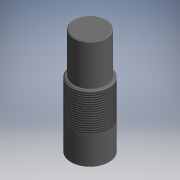
# Autodesk Inventor part: ESBF-BS-100-ESBF-BS-100---(KSA)
Saved by Autodesk Inventor 2017.3 (Build 213256000, 256)
## iProperties
Part Number: ESBF-BS-100-ESBF-BS-100---(KSA)
Material: Generic
Catalog Web Link: www.cadenas.de
Description: ESBF-(KSA)-Electro-cylinder
Vendor: FESTO
Document SubType Name: Modeling
Designer: partserver
Manufacturer: FESTO
Mass: 43.39 g
Surface Area: 76.8882 cm^2
Volume: 43.39 cm^3
Density: 1 g/cm^3
Appearance: PSOLRGB-128-128-128
Category: PARTsolutions
Company: FESTO
Title: ESBF-BS-100-ESBF-BS-100---(KSA)
Author: Cadenas PARTsolutions
Comments: Electro-cylinder
PSOL_IDENT_0: {$CADENAS_DATA\23d-libs\festo\parts\e\esbf\parts\esbf_ksa.prj},206 {VTYP=3D},{NB=ESBF-BS-100-ESBF-BS
PSOL_IDENT_1: -100---(KSA)},{LINA=ESBF-BS-100-ESBF-BS-100---(KSA)},{NN=ESBF-(KSA)},{DATE=13.05.2020 13:32:49},{GEO
PSOL_IDENT_2: MDATE=02.09.2015 14:29:35},{VERSION=},{LINEID=30},{WBVAR=},{WBNUMERIC=}  {NB=ESBF-BS-100-ESBF-BS-100
PSOL_IDENT_3: ---(KSA)},{LINA=ESBF-BS-100-ESBF-BS-100---(KSA)},{KT=DUMMY},{TNR=574092},{TYP=ESBF-BS-100},{KDM=100}
PSOL_IDENT_4: ,{D2=24.000},{L3=39.500},{L4=30.000},{G=39.000},{G1=39.000},{GUA=28.000},{P=1.500}
NB: ESBF-BS-100-ESBF-BS-100---(KSA)
NN: ESBF-(KSA)
NT: Electro-cylinder
NBSYN: $TYP.-$TYP.---(KSA)
LINA: ESBF-BS-100-ESBF-BS-100---(KSA)
CATALOG: Festo
TNR: 574092
TYP: ESBF-BS-100
KDM: 100
D2: 24
L3: 39.5
L4: 30
G: 39
G1: 39
GUA: 28
P: 1.5
SUPPLIER: FESTO
ARTICLENO: ESBF-BS-100-ESBF-BS-100---(KSA)
BOMINFO: ESBF-BS-100-ESBF-BS-100---(KSA)
CREATOR: CADENAS GmbH
Autodesk Inventor part; units mm, degrees
sketch "Sketch_1" plane through (0, 0, 0) normal (1, 0, 0) x (0, 1, 0)
  line L0 (0, -78.5) -> (0, 0)
  line L1 (0, 0) -> (14, 0)
  line L2 (14, 0) -> (14, -47.58)
  line L3 (14, -47.58) -> (13.08, -48.5)
  line L4 (13.08, -48.5) -> (12, -48.5)
  line L5 (12, -48.5) -> (12, -78)
  line L6 (12, -78) -> (11.5, -78.5)
  line L7 (11.5, -78.5) -> (0, -78.5)
  line L8 (0, -78.5) -> (0, 0)
  constraints: 18 end point
revolve "Revolution1" add sketch "Sketch_1" angle 360 about axis through (0, 0, -78.5) along (0, 0, -1)
thread "Thread1" size "M28x1.5" class "6g" standard "ISO Metric profile" length 27.08
ref_plane "ANBAU_XY" through (0, 0, 0) normal (0, 0, 1) x (1, 0, 0)
ref_plane "ANBAU_YZ" through (0, 0, 0) normal (1, 0, 0) x (0, 1, 0)
ref_plane "ANBAU_ZX" through (0, 0, 0) normal (0, 1, 0) x (0, 0, 1)
body "Solid1"
